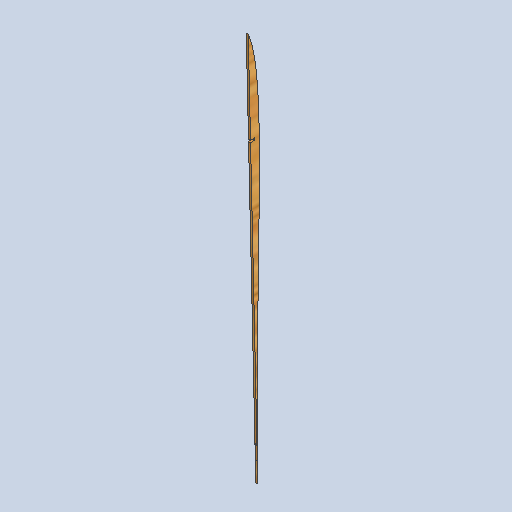
# Autodesk Inventor part: standoff
Saved by Autodesk Inventor 2022 (Build 260153070, 153G)
## iProperties
Created: 2021-05-01
Part Number: standoff
Material: Plywood, Sheathing, Glazed
Document SubType Name: Modeling
Designer: kardo
Density: 0.75 g/cm^3
Appearance: Plywood - New(2)
Mass: 2.72628 g
Surface Area: 52.2476 cm^2
Volume: 3.63504 cm^3
Author: kardo
Autodesk Inventor part; units mm, degrees
ref_plane "YZ Plane" through (0, 0, 0) normal (1, 0, 0) x (0, 1, 0)
ref_plane "XZ Plane" through (0, 0, 0) normal (0, 1, 0) x (-1, 0, 0)
ref_plane "XY Plane" through (0, 0, 0) normal (0, 0, 1) x (1, 0, 0)
derived "frame_outline.ipt"
sketch "standoff" plane through (30, 0, 0) normal (1, 0, 0) x (0, 1, 0)
  line L0 (94.8, 28.832) -> (28.4595, 27.2216)
  line L1 (28.4595, 27.2216) -> (-37.9005, 25.6108)
  line L2 (-37.9005, 25.6108) -> (-277.6703, 19.7906)
  line L3 (-363, 18.496) -> (-297.6664, 19.4083)
  spline S0 degree 4 poles (-297.6664, 19.4083) (-178.2238, 21.0761) (-46.6271, 18.3209) (53.0846, 11.363) (94.8, 28.832) knots 0 0 0 0 0 1 1 1 1 1
  spline S1 degree 3 poles (-297.6664, 19.4083) (-291.0004, 19.5014) (-284.3349, 19.6288) (-277.6703, 19.7906) knots 0 0 0 0 1 1 1 1
  point P0 (0, 0)
extrude "Extrusion1" add sketch "standoff" against normal blind 2
sketch "Sketch2" plane through (30, -101.4011, 21.3607) normal (1, 0, 0) x (0, 0.3862654, -0.9223877)
  line L0 (-149.7634, 172.6492) -> (228.0988, 14.413) projected
  line L1 (38.3958, 93.8544) -> (39.1683, 95.6991)
  line L2 (39.1683, 95.6991) -> (35.1266, 97.3917)
  line L3 (-66.6384, -163.195) -> (68.8943, 183.8594) projected
  point P0 (58.8706, 85.2802)
  point P1 (34.3989, 95.5281)
  point P2 (42.3927, 92.1806)
  dimension "d3" = 2
  constraints: 5 point on line, 4 end point, 1 parallel, 1 perpendicular, 1 symmetric about line, 2 other
  measures "d3" distance between parallel lines of L0 L2
extrude "Extrusion2" cut sketch "Sketch2" against normal through all
equation "\"d1\" = bulkhead_thickness"
equation "\"d3\" = bulkhead_thickness"
equation "\"bulkhead_thickness\" = 2"
body "Solid1"
